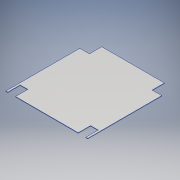
# Autodesk Inventor part: BK-BKT120-BasePlateextruded
Saved by Autodesk Inventor 2017 (Build 210142000, 142)
## iProperties
Created: 2016-09-24
Part Number: BK-BKT120-BasePlateextruded
Material: Aluminum 6061
Document SubType Name: Modeling
Designer: vslabsal
Density: 2.7 g/cm^3
Appearance: Aluminum - Flat
Author: vslabsal
Autodesk Inventor part; units mm, degrees
ref_plane "YZ Plane" through (0, 0, 0) normal (1, 0, 0) x (0, 1, 0)
ref_plane "XZ Plane" through (0, 0, 0) normal (0, 1, 0) x (-1, 0, 0)
ref_plane "XY Plane" through (0, 0, 0) normal (0, 0, 1) x (1, 0, 0)
sketch "Sketch1" plane through (0, 0, 0) normal (0, 0, 1) x (1, 0, 0)
  line L0 (270.51, 284.48) -> (-270.51, -284.48) construction
  line L1 (-270.51, 284.48) -> (270.51, -284.48) construction
  line L2 (-270.51, -284.48) -> (-257.81, -284.48)
  line L3 (-257.81, -284.48) -> (-257.81, -203.2)
  line L4 (-257.81, -203.2) -> (-207.01, -203.2)
  line L5 (-207.01, -203.2) -> (-207.01, -284.48)
  line L6 (-207.01, -284.48) -> (207.01, -284.48)
  line L7 (207.01, -284.48) -> (207.01, -203.2)
  line L8 (207.01, -203.2) -> (257.81, -203.2)
  line L9 (257.81, -203.2) -> (257.81, -284.48)
  line L10 (257.81, -284.48) -> (270.51, -284.48)
  line L11 (270.51, -284.48) -> (270.51, 203.2)
  line L12 (270.51, 203.2) -> (207.01, 203.2)
  line L13 (207.01, 203.2) -> (207.01, 284.48)
  line L14 (207.01, 284.48) -> (-207.01, 284.48)
  line L15 (-207.01, 203.2) -> (-207.01, 284.48)
  line L16 (-207.01, 203.2) -> (-270.51, 203.2)
  line L17 (-270.51, 203.2) -> (-270.51, -284.48)
  point P0 (0, 0)
  point P1 (0, 0)
  dimension "d0" = 541.02
  dimension "d1" = 568.96
  dimension "d2" = 12.7
  dimension "d3" = 81.28
  dimension "d4" = 50.8
  dimension "d5" = 81.28
  dimension "d6" = 414.02
  dimension "d7" = 81.28
  dimension "d8" = 50.8
  dimension "d9" = 81.28
  dimension "d10" = 12.7
  dimension "d11" = 487.68
  dimension "d12" = 63.5
  dimension "d13" = 81.28
  dimension "d14" = 414.02
  dimension "d15" = 81.28
  dimension "d16" = 63.5
  constraints: 36 end point, 8 horizontal, 8 vertical, 2 midpoint, 2 point on line
  measures "d0" distance of L0.end L1.end
  measures "d1" distance of L1.start L0.end
  measures "d2" distance of L0.end L2.end
  measures "d3" distance of L2.end L3.end
  measures "d4" distance of L3.end L4.end
  measures "d5" distance of L4.end L5.end
  measures "d6" distance of L5.end L6.end
  measures "d7" distance of L7.start L7.end
  measures "d8" distance of L7.end L8.end
  measures "d9" distance of L8.end L9.end
  measures "d10" distance of L9.end L1.end
  measures "d11" distance of L1.end L11.end
  measures "d12" distance of L11.end L12.end
  measures "d13" distance of L12.end L13.end
  measures "d14" distance of L14.end L13.end
  measures "d15" distance of L15.start L14.end
  measures "d16" distance of L16.start L16.end
extrude "Extrusion1" add sketch "Sketch1" along normal blind 3.175
body "Solid1"
